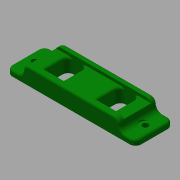
# Autodesk Inventor part: SingleRegulatorSupport
Saved by Autodesk Inventor 2014 (Build 180170000, 170)
## iProperties
Created: 2015-07-07
Part Number: SingleRegulatorSupport
Material: Generic
Document SubType Name: Modeling
Designer: Karl
Density: 1 g/cm^3
Appearance: Dark Green
Author: Karl
Autodesk Inventor part; units mm, degrees
ref_plane "YZ Plane" through (0, 0, 0) normal (1, 0, 0) x (0, 1, 0)
ref_plane "XZ Plane" through (0, 0, 0) normal (0, 1, 0) x (-1, 0, 0)
ref_plane "XY Plane" through (0, 0, 0) normal (0, 0, 1) x (1, 0, 0)
sketch "Sketch1" plane through (0, 0, 0) normal (0, 1, 0) x (-1, 0, 0)
  line L0 (36.83, -10.795) -> (-36.83, -10.795)
  line L1 (-36.83, -10.795) -> (-36.83, 10.795)
  line L2 (-36.83, 10.795) -> (36.83, 10.795)
  line L3 (36.83, 10.795) -> (36.83, -10.795)
  line L4 (36.83, -10.795) -> (-36.83, 10.795) construction
  line L5 (-36.83, -10.795) -> (36.83, 10.795) construction
  point P0 (0, 0)
  dimension "d0" = 21.59
  dimension "d1" = 73.66
  constraints: 12 end point, 2 midpoint, 2 parallel, 1 horizontal, 1 perpendicular
  measures "d0" distance of L0.end L1.end
  measures "d1" distance of L1.end L2.end
extrude "Extrusion1" add sketch "Sketch1" along normal blind 9.525
sketch "Sketch2" plane through (0, 9.525, 0) normal (0, 1, 0) x (1, 0, 0)
  line L0 (36.83, 10.795) -> (-36.83, 10.795) projected
  line L1 (27.559, -10.795) -> (-27.559, -10.795)
  line L2 (-27.559, -10.795) -> (-27.559, 10.795)
  line L3 (-27.559, 10.795) -> (27.559, 10.795)
  line L4 (27.559, 10.795) -> (27.559, -10.795)
  line L5 (27.559, -10.795) -> (-27.559, 10.795) construction
  line L6 (-27.559, -10.795) -> (27.559, 10.795) construction
  line L7 (-36.83, 10.795) -> (-27.559, 10.795)
  line L8 (-27.559, 10.795) -> (-27.559, -10.795)
  line L9 (-27.559, -10.795) -> (-36.83, -10.795)
  line L10 (-36.83, -10.795) -> (-36.83, 10.795)
  line L11 (27.559, 10.795) -> (36.83, 10.795)
  line L12 (36.83, 10.795) -> (36.83, -10.795)
  line L13 (36.83, -10.795) -> (27.559, -10.795)
  line L14 (27.559, -10.795) -> (27.559, 10.795)
  point P0 (0, 0)
  dimension "d4" = 55.118
  constraints: 28 end point, 6 parallel, 3 horizontal, 3 perpendicular, 2 midpoint, 1 collinear
  measures "d4" distance of L2.end L3.end
extrude "Extrusion2" cut sketch "Sketch2" against normal blind 6.35 contours L12 L13 L4 L0 | L2 L9 L10 L0
sketch "Sketch3" plane through (0, 9.525, 0) normal (0, 1, 0) x (1, 0, 0)
  line L0 (-27.559, 10.795) -> (-27.559, -10.795) projected
  line L1 (27.559, -7.8105) -> (-27.559, -7.8105)
  line L2 (-27.559, -7.8105) -> (-27.559, 7.8105)
  line L3 (-27.559, 7.8105) -> (27.559, 7.8105)
  line L4 (27.559, 7.8105) -> (27.559, -7.8105)
  line L5 (27.559, -7.8105) -> (-27.559, 7.8105) construction
  line L6 (-27.559, -7.8105) -> (27.559, 7.8105) construction
  point P0 (0, 0)
  dimension "d7" = 15.621
  constraints: 12 end point, 2 midpoint, 2 parallel, 1 collinear, 1 horizontal, 1 perpendicular
  measures "d7" distance of L1.end L2.end
extrude "Extrusion3" cut sketch "Sketch3" against normal blind 1.651
sketch "Sketch4" plane through (0, 7.874, 0) normal (0, 1, 0) x (1, 0, 0)
  line L0 (27.559, -7.8105) -> (-27.559, -7.8105) projected
  line L1 (27.559, 7.8105) -> (27.559, -7.8105) projected
  line L2 (-27.559, 7.8105) -> (27.559, 7.8105) projected
  line L3 (-27.559, -7.8105) -> (-27.559, 7.8105) projected
  line L4 (-20.32, 7.8105) -> (-9.525, 7.8105)
  line L5 (-9.525, 7.8105) -> (-9.525, -7.8105)
  line L6 (-9.525, -7.8105) -> (-20.32, -7.8105)
  line L7 (-20.32, -7.8105) -> (-20.32, 7.8105)
  line L8 (9.525, 7.8105) -> (20.32, 7.8105)
  line L9 (20.32, 7.8105) -> (20.32, -7.8105)
  line L10 (20.32, -7.8105) -> (9.525, -7.8105)
  line L11 (9.525, -7.8105) -> (9.525, 7.8105)
  point P0 (0, 0)
  dimension "d10" = 7.239
  dimension "d11" = 9.525
  dimension "d12" = 7.239
  dimension "d13" = 9.525
  constraints: 16 end point, 4 parallel, 4 point on line, 2 horizontal, 2 perpendicular
  measures "d10" distance between parallel lines of L3 L7
  measures "d11" distance from line of L5 point (0, 0)
  measures "d12" distance between parallel lines of L1 L9
  measures "d13" distance from line of point (0, 0) L11
extrude "Extrusion4" cut sketch "Sketch4" against normal blind 25.4 contours L0 L11 L2 L9 | L0 L7 L2 L5
sketch "Sketch5" plane through (0, 3.175, 0) normal (0, 1, 0) x (1, 0, 0)
  line L0 (-36.83, -10.795) -> (-36.83, 10.795) projected
  line L1 (-27.559, -10.795) -> (-36.83, -10.795) projected
  line L2 (-27.559, 10.795) -> (-27.559, -10.795) projected
  line L3 (-36.83, 10.795) -> (-27.559, 10.795) projected
  point P0 (0, 0)
  point P1 (-31.75, 0)
  point P2 (31.75, 0)
  dimension "d16" = 31.75
  dimension "d17" = 31.75
  constraints: 2 horizontal alignment
  measures "d16" distance of point (0, 0) point (-31.75, 0)
  measures "d17" distance of point (31.75, 0) point (0, 0)
hole "Hole1" at (-31.75, 3.175, 0) at (31.75, 3.175, 0) direction (0, -1, 0) diameter 3.302 depth 25.4 tip angle 118
fillet "Fillet1" radius 3.175 6 edges at (36.83, 1.5875, 10.795) (36.83, 1.5875, -10.795) (-36.83, 1.5875, 10.795) (-36.83, 1.5875, -10.795) (-27.559, 3.175, 0) (27.559, 3.175, 0)
fillet "Fillet2" radius 3.175 2 edges at (-27.559, 9.525, -9.3027) (27.559, 9.525, -9.3028)
fillet "Fillet3" radius 3.175 8 edges at (-9.525, 3.937, -7.8105) (20.32, 3.937, -7.8105) (9.525, 3.937, -7.8105) (-9.525, 3.937, 7.8105) (-20.32, 3.937, 7.8105) (-20.32, 3.937, -7.8105) (9.525, 3.937, 7.8105) (20.32, 3.937, 7.8105)
fillet "Fillet4" radius 1.27 36 edges at (26.6292, 8.5952, 10.795) (27.559, 6.3502, 10.795) (28.4889, 4.1049, 10.795) (32.1945, 3.175, 10.795) (35.9001, 3.175, 9.8651) (36.83, 3.175, 0) (35.9001, 3.175, -9.8651) (32.1945, 3.175, -10.795) (28.4889, 4.1049, -10.795) (26.6292, 8.5952, -10.795) (27.559, 6.3502, -10.795) (0.0001, 9.525, -10.795) (-26.6291, 8.5951, -10.795) (-27.559, 6.3501, -10.795) (-28.4889, 4.1049, -10.795) (-32.1945, 3.175, -10.795) (-35.9001, 3.175, -9.8651) (-36.83, 3.175, 0) (-35.9001, 3.175, 9.8651) (-32.1945, 3.175, 10.795) (-27.559, 6.3501, 10.795) (-28.4889, 4.1049, 10.795) (-26.6291, 8.5951, 10.795) (0.0001, 9.525, 10.795) (10.4549, 7.874, -6.8806) (10.4549, 7.874, 6.8806) (9.525, 7.874, 0) (19.3901, 7.874, 6.8806) (19.3901, 7.874, -6.8806) (20.32, 7.874, 0) (-10.4549, 7.874, 6.8806) (-10.4549, 7.874, -6.8806) (-9.525, 7.874, 0) (-19.3901, 7.874, -6.8806) (-19.3901, 7.874, 6.8806) (-20.32, 7.874, 0)
sketch "Sketch6" plane through (0, 3.175, 0) normal (0, 1, 0) x (1, 0, 0)
  arc A0 (-30.734, 1.3014) -> (-30.734, -1.3014) centre (-31.75, 0) ccw projected
  arc A1 (30.734, -1.3014) -> (30.734, 1.3014) centre (31.75, 0) ccw projected
  circle A2 centre (-31.75, 0) radius 3.175
  circle A3 centre (31.75, 0) radius 3.175
  point P0 (0, 0)
  dimension "d29" = 6.35
  dimension "d30" = 6.35
  constraints: 2 centre point, 2 coincident
  measures "d29" diameter of A2
  measures "d30" diameter of A3
extrude "Extrusion5" cut sketch "Sketch6" along normal blind 25.4
body "Solid1"
